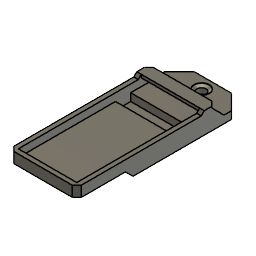
SolarSensor_Mount (Autodesk Fusion 360 design; units mm, degrees)
part number: 2026-03-04-11-55-40-864
Autodesk Fusion 360 part; units mm, degrees
sketch "Sketch1" plane through (0, 0, 0) normal (0, 1, 0) x (1, 0, 0)
  line L0 (0, 0) -> (38.5, 0)
  line L1 (0, 0) -> (0, -86)
  line L2 (0, -86) -> (38.5, -86)
  line L3 (38.5, -86) -> (38.5, 0)
  line L4 (38.5, 0) -> (0, 0)
  line L5 (0, 0) -> (0, -86)
  line L6 (0, 0) -> (-3, 0)
  line L7 (-3, 0) -> (-3, 3)
  line L8 (-3, 3) -> (0, 3)
  line L9 (0, 3) -> (0, 0)
  line L10 (38.5, -86) -> (41.5, -86)
  line L11 (41.5, -86) -> (41.5, -89)
  line L12 (41.5, -89) -> (38.5, -89)
  line L13 (38.5, -89) -> (38.5, -86)
  line L14 (41.5, -89) -> (-3, -89)
  line L15 (-3, -89) -> (-3, 3)
  line L16 (-3, 3) -> (41.5, 3)
  line L17 (41.5, 3) -> (41.5, -89)
  dimension "d1" = 38.5
  dimension "d2" = 86
  dimension "d3" = 3
  dimension "d4" = 3
  dimension "d5" = 3
  dimension "d6" = 3
  constraint coincident L0.start L1.start
  constraint horizontal L0
  constraint perpendicular L0 L1
  constraint horizontal L2
  constraint vertical L3
  constraint horizontal L4
  constraint vertical L5
  constraint horizontal L6
  constraint vertical L7
  constraint horizontal L8
  constraint vertical L9
  constraint horizontal L10
  constraint vertical L11
  constraint horizontal L12
  constraint vertical L13
  constraint horizontal L14
  constraint vertical L15
  constraint horizontal L16
  constraint vertical L17
  measures "d1" distance of L0.start L0.end
  measures "d2" distance of L0.start L1.end
  measures "d3" distance of L0.start L6.end
  measures "d4" distance of L0.start L8.end
  measures "d5" distance of L2.end L10.end
  measures "d6" distance of L2.end L12.end
extrude "Extrude1" add sketch "Sketch1" against normal blind 2
extrude "Extrude2" add sketch "Sketch1" along normal blind 5 contours L0 L3 L4 L9 L10 L16 L17 | L1 L2 L5 L6 L13 L14 L15 | L6 L7 L8 L9 L15 L16 | L10 L11 L12 L13 L14 L17
sketch "Sketch2" plane through (0, 0, 0) normal (0, 1, 0) x (-1, 0, 0)
  line L0 (0, 86) -> (-38.5, 86)
  line L1 (-38.5, 86) -> (-38.5, 0)
  line L2 (-38.5, 0) -> (0, 0)
  line L3 (0, 0) -> (0, 86)
  line L4 (0, 0) -> (0, 12)
  line L5 (0, 12) -> (-38.5, 12)
  line L6 (-38.5, 12) -> (-38.5, 22)
  line L7 (-38.5, 22) -> (0, 22)
  line L8 (0, 22) -> (0, 12)
  dimension "d11" = 12
  dimension "d12" = 10
  constraint coincident L2.end L3.start
  constraint perpendicular L2 L4
  constraint horizontal L5
  constraint vertical L6
  constraint horizontal L7
  constraint vertical L8
  measures "d11" distance of L2.end L4.end
  measures "d12" distance of L4.end L7.end
extrude "Extrude3" cut sketch "Sketch2" against normal blind 5 contours L1 L3 L5 L6 L7 L8
sketch "Sketch3" plane through (0, 5, 0) normal (0, 1, 0) x (-1, 0, 0)
  line L0 (0, 86) -> (0, 0)
  line L1 (0, 0) -> (-38.5, 0)
  line L2 (-38.5, 0) -> (-38.5, 86)
  line L3 (-38.5, 86) -> (0, 86)
  line L4 (-41.5, -3) -> (3, -3)
  line L5 (3, -3) -> (3, 89)
  line L6 (3, 89) -> (-41.5, 89)
  line L7 (-41.5, 89) -> (-41.5, -3)
  line L8 (-38.5, 0) -> (-38.5, 5)
  line L9 (-38.5, 5) -> (-41.5, 5)
  line L10 (-38.5, 5) -> (3, 5)
  dimension "d15" = 5
  constraint coincident L1.end L2.start
  constraint perpendicular L1 L8
  constraint coincident L7 L9.end
  constraint perpendicular L7 L9
  constraint coincident L5 L10.end
  constraint perpendicular L5 L10
  measures "d15" distance of L1.end L8.end
extrude "Extrude4" add sketch "Sketch3" along normal blind 2 contours L0 L1 L2 L4 L5 L7 L8 L9 L10 | L0 L1 L2 L8 L10
fillet "Fillet1" radius 5 1 edges at (19.25, 5, 0)
sketch "Sketch4" plane through (0, -2, 0) normal (0, -1, 0) x (1, 0, 0)
  line L0 (38.5, 22) -> (38.5, 12)
  line L1 (38.5, 12) -> (0, 12)
  line L2 (0, 12) -> (0, 22)
  line L3 (0, 22) -> (38.5, 22)
  line L4 (-3, -3) -> (41.5, -3)
  line L5 (41.5, -3) -> (41.5, 89)
  line L6 (41.5, 89) -> (-3, 89)
  line L7 (-3, 89) -> (-3, -3)
  line L8 (0, 12) -> (-3, 12)
  line L9 (-3, 12) -> (-3, 9)
  line L10 (-3, 9) -> (0, 9)
  line L11 (0, 9) -> (0, 12)
  line L12 (38.5, 22) -> (41.5, 22)
  line L13 (41.5, 22) -> (41.5, 52)
  line L14 (41.5, 52) -> (38.5, 52)
  line L15 (38.5, 52) -> (38.5, 22)
  line L16 (41.5, 52) -> (-3, 52)
  line L17 (-3, 52) -> (-3, 9)
  line L18 (41.5, 9) -> (41.5, 52)
  line L19 (0, 22) -> (0, 52)
  line L20 (0, 22) -> (5, 22)
  line L21 (5, 22) -> (0, 22)
  line L22 (0, 22) -> (0, 52)
  line L23 (0, 52) -> (5, 52)
  line L24 (5, 52) -> (5, 22)
  line L25 (-3, -3) -> (-3, -23)
  line L26 (-3, -23) -> (41.5, -23)
  line L27 (41.5, -23) -> (41.5, -3)
  line L28 (41.5, -3) -> (-3, -3)
  line L29 (-3, -3) -> (-3, -23)
  dimension "d20" = 3
  dimension "d21" = 30
  dimension "d29" = 5
  dimension "d45" = 20
  constraint horizontal L8
  constraint vertical L9
  constraint horizontal L10
  constraint vertical L11
  constraint coincident L1.end L2.start
  constraint horizontal L12
  constraint vertical L13
  constraint horizontal L14
  constraint vertical L15
  constraint coincident L0.start L3.end
  constraint horizontal L16
  constraint vertical L17
  constraint vertical L18
  constraint coincident L2.end L3.start
  constraint coincident L16 L19.end
  constraint perpendicular L16 L19
  constraint perpendicular L19 L20
  constraint horizontal L21
  constraint vertical L22
  constraint horizontal L23
  constraint vertical L24
  constraint coincident L4.start L7.end
  constraint perpendicular L4 L25
  constraint horizontal L26
  constraint vertical L27
  constraint horizontal L28
  constraint vertical L29
  constraint coincident L4.end L5.start
  measures "d20" distance of L1.end L10.end
  measures "d21" distance of L0.start L14.end
  measures "d29" distance of L2.end L20.end
  measures "d45" distance of L4.start L25.end
extrude "Extrude5" add sketch "Sketch4" along normal blind 5 contours L0 L1 L4 L5 L7 L10 L11 L12 L18 L28 | L5 L12 L13 L14 L15 L16 L18 | L3 L15 L16 L24 | L2 L7 L8 L16 L17 L19 L22 | L7 L8 L9 L10 L11 L17 | L4 L25 L26 L27 L28 L29
sketch "Sketch5" plane through (0, 0, 0) normal (0, 1, 0) x (-1, 0, 0)
  line L0 (-38.5, 22) -> (0, 22)
  line L1 (0, 22) -> (0, 86)
  line L2 (0, 86) -> (-38.5, 86)
  line L3 (-38.5, 86) -> (-38.5, 22)
  line L4 (0, 86) -> (-10, 86)
  line L5 (-38.5, 86) -> (-28.5, 86)
  line L6 (-28.5, 86) -> (-28.5, 81)
  line L7 (-28.5, 81) -> (-10, 81)
  line L8 (-10, 81) -> (-10, 86)
  line L9 (-10, 86) -> (-28.5, 86)
  line L10 (-28.5, 86) -> (-28.5, 81)
  dimension "d24" = 10
  dimension "d25" = 10
  dimension "d26" = 5
  constraint coincident L1.end L2.start
  constraint perpendicular L1 L4
  constraint coincident L2.end L3.start
  constraint perpendicular L3 L5
  constraint perpendicular L5 L6
  constraint horizontal L7
  constraint vertical L8
  constraint horizontal L9
  constraint vertical L10
  measures "d24" distance of L1.end L4.end
  measures "d25" distance of L2.end L5.end
  measures "d26" distance of L5.end L6.end
extrude "Extrude6" cut sketch "Sketch5" against normal blind 2 contours L2 L6 L7 L8 L9 L10
sketch "Sketch6" plane through (0, -7, 0) normal (0, -1, 0) x (1, 0, 0)
  line L0 (5, 52) -> (5, 22)
  line L1 (5, 22) -> (38.5, 22)
  line L2 (38.5, 22) -> (38.5, 12)
  line L3 (38.5, 12) -> (0, 12)
  line L4 (0, 12) -> (0, 52)
  line L5 (0, 52) -> (-3, 52)
  line L6 (-3, 52) -> (-3, -23)
  line L7 (41.5, -23) -> (41.5, 52)
  line L8 (41.5, 52) -> (5, 52)
  line L9 (5, 22) -> (0, 22)
  line L10 (0, 32) -> (5, 32)
  line L11 (-3, -23) -> (41.5, -23)
  constraint coincident L0.end L1.start
  constraint coincident L4 L9.end
  constraint perpendicular L4 L9
  constraint midpoint L4 L10.start
  constraint coincident L0 L10.end
  constraint perpendicular L0 L10
extrude "Extrude7" add sketch "Sketch6" against normal blind 2 contours L0 L4 L9 L10 | L1 L2 L3 L4 L9
fillet "Fillet2" radius 2.5 2 edges at (5, -2, 37) (0, -2, 37)
chamfer "Chamfer1" distance 5 angle 45 3 edges at (22, -2, 52) (-0.25, -2, 52) (19.25, -2, -3) tangent chain off
chamfer "Chamfer2" distance 3 angle 45 4 edges at (41.5, 1.5, 89) (41.5, 5, -3) (-3, 5, -3) (-3, 1.5, 89) tangent chain off
chamfer "Chamfer3" distance 2 angle 45 2 edges at (-1.5, 5, 5) (40, 5, 5) tangent chain off
chamfer "Chamfer4" distance 10 angle 45 2 edges at (41.5, -4.5, -23) (-3, -4.5, -23) tangent chain off
sketch "Sketch9" plane through (0, -2, 0) normal (0, 1, 0) x (-1, 0, 0)
  line L0 (-7, -23) -> (3, -13)
  line L1 (3, -13) -> (3, -8)
  line L2 (3, -8) -> (-41.5, -8)
  line L3 (-41.5, -8) -> (-41.5, -13)
  line L4 (-41.5, -13) -> (-31.5, -23)
  line L5 (-31.5, -23) -> (-7, -23)
  line L6 (-19.25, -23) -> (-19.25, -8)
  circle A0 centre (-19.25, -15.5) radius 3
  dimension "d47" = 6
  constraint midpoint L5 L6.start
  constraint midpoint L2 L6.end
  constraint midpoint L6 A0.centre
  measures "d47" diameter of A0
extrude "Extrude10" cut sketch "Sketch9" against normal blind 10 contours L6 A0 | L6 A0
hole "Hole2" at (19.25, -2, -15.5) direction (0, -1, 0) diameter 10 depth 0.2 tip angle 118
named bodies: "SolarSensorMount"
